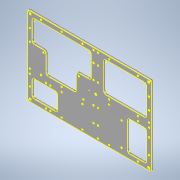
# Autodesk Inventor part: Platta
Saved by Autodesk Inventor 2021 (Build 250183000, 183)
## iProperties
Created: 2020-02-23
Part Number: Platta
Material: Generic
Document SubType Name: Modeling
Designer: lgnds
Density: 1 g/cm^3
Appearance: Default
Author: lgnds
Autodesk Inventor part; units mm, degrees
ref_plane "YZ Plane" through (0, 0, 0) normal (1, 0, 0) x (0, 1, 0)
ref_plane "XZ Plane" through (0, 0, 0) normal (0, 1, 0) x (-1, 0, 0)
ref_plane "Work Plane1" through (-121.526, 76.2535, 6) normal (0, 0, 1) x (1, 0, 0)
sketch "Sketch1" plane through (-121.526, 76.2535, 6) normal (0, 0, 1) x (1, 0, 0)
  line L0 (-3.6706, 3.4431) -> (246.7225, 3.4431)
  line L1 (246.7225, 3.4431) -> (246.7225, -155.95)
  line L2 (246.7225, -155.95) -> (-3.6706, -155.95)
  line L3 (-3.6706, -155.95) -> (-3.6706, 3.4431)
  line L4 (247.7225, -156.2501) -> (247.7225, 3.7432) projected
  line L5 (247.0226, -156.75) -> (-3.9707, -156.75) construction
  line L6 (247.0226, -156.75) -> (-3.9707, -156.75) projected
  line L7 (247.0226, 4.4431) -> (-3.9707, 4.4431) projected
  line L8 (247.0297, -157.8069) -> (-3.9777, -157.8069) projected
  ellipse E0 centre (247.0292, -156.2567) end of major axis (248.1256, -157.353) minor radius 1.55 (247.0297, -157.8069) -> (248.5794, -156.2572) ccw projected
  line L9 (248.5794, 3.7502) -> (248.5794, -156.2572) projected
  ellipse E1 centre (247.0292, 3.7498) end of major axis (248.1256, 4.8461) minor radius 1.55 (248.5794, 3.7502) -> (247.0297, 5.3) ccw projected
  line L10 (-3.9777, 5.3) -> (247.0297, 5.3) projected
  line L11 (-5.5275, -156.2572) -> (-5.5275, 3.7502) projected
  ellipse E2 centre (-3.9772, -156.2567) end of major axis (-5.0736, -157.353) minor radius 1.55 (-5.5275, -156.2572) -> (-3.9777, -157.8069) ccw projected
  ellipse E3 centre (-3.9705, 3.743) end of major axis (-4.4656, 4.2381) minor radius 0.7 (-3.9707, 4.4431) -> (-4.6706, 3.7432) ccw projected
  line L12 (247.0226, 4.4431) -> (-3.9707, 4.4431) projected
  ellipse E4 centre (247.0224, 3.743) end of major axis (247.5175, 4.2381) minor radius 0.7 (247.7225, 3.7432) -> (247.0226, 4.4431) ccw projected
  line L13 (247.7225, -156.2501) -> (247.7225, 3.7432) projected
  ellipse E5 centre (247.0224, -156.2499) end of major axis (247.5175, -156.745) minor radius 0.7 (247.0226, -156.95) -> (247.7225, -156.2501) ccw projected
  line L14 (-3.9707, -156.95) -> (247.0226, -156.95) projected
  line L15 (-4.6706, 3.7432) -> (-4.6706, -156.2501) projected
  line L16 (237.7225, -5.5569) -> (5.3294, -5.5569)
  line L17 (5.3294, -5.5569) -> (5.3294, -146.95)
  line L18 (5.3294, -146.95) -> (237.7225, -146.95)
  line L19 (237.7225, -146.95) -> (237.7225, -5.5569)
  ellipse E6 centre (-3.9772, 3.7498) end of major axis (-5.0736, 4.8461) minor radius 1.55 (-3.9777, 5.3) -> (-5.5275, 3.7502) ccw projected
  ellipse E7 centre (-3.9705, -156.2499) end of major axis (-4.4656, -156.745) minor radius 0.7 (-4.6706, -156.2501) -> (-3.9707, -156.95) ccw projected
  point P0 (121.526, -76.2535)
  dimension "d0" = 1
  dimension "d1" = 1
  dimension "d2" = 1
  dimension "d3" = 1
  dimension "d4" = 9
  constraints: 16 end point, 4 parallel, 2 perpendicular, 1 horizontal, 11 other
  measures "d0" distance between parallel lines of L7 L0
  measures "d1" distance between parallel lines of L15 L3
  measures "d2" distance between parallel lines of L4 L1
  measures "d3" distance between parallel lines of L14 L2
  measures "d4" distance between parallel lines of L0 L16
extrude "Extrusion1" add sketch "Sketch1" along normal blind 2.9864 contours L0 L1 L2 L3
sketch "Sketch2" plane through (-121.526, 76.2535, 8.9864) normal (0, 0, 1) x (1, 0, 0)
  circle A0 centre (1.526, -1.2535) radius 1.621 construction
  circle A1 centre (1.526, -151.2535) radius 1.621 construction
  circle A2 centre (241.526, -151.2535) radius 2.121 construction
  circle A3 centre (241.526, -1.2535) radius 2.121 construction
  circle A4 centre (1.526, -1.2535) radius 2.1
  line L0 (-92.7978, -76.2535) -> (335.0689, -76.2535) construction
  line L1 (121.526, -201.3727) -> (121.526, 48.8923) construction
  circle A5 centre (1.526, -151.2535) radius 1.621 construction
  circle A6 centre (1.526, -151.2535) radius 2.1
  circle A7 centre (241.526, -1.2535) radius 1.621 construction
  circle A8 centre (241.526, -151.2535) radius 1.621 construction
  circle A9 centre (241.526, -1.2535) radius 2.1
  circle A10 centre (241.526, -151.2535) radius 1.621 construction
  circle A11 centre (241.526, -151.2535) radius 2.1
  point P0 (121.526, -76.2535)
  point P1 (335.8498, -76.2535)
  dimension "d9" = 4.2
  constraints: 8 centre point, 8 symmetric about line, 4 coincident, 4 end point, 1 horizontal, 1 vertical, 11 other
  measures "d9" diameter of A4
extrude "Extrusion2" cut sketch "Sketch2" against normal up to next
sketch "Sketch3" plane through (-121.526, 76.2535, 8.9864) normal (0, 0, 1) x (1, 0, 0)
  line L0 (335.0689, -76.2535) -> (-92.7978, -76.2535) construction
  line L1 (5.3294, -81.2535) -> (237.7225, -81.2535)
  line L2 (237.7225, -81.2535) -> (237.7225, -71.2535)
  line L3 (237.7225, -71.2535) -> (5.3294, -71.2535)
  line L4 (5.3294, -71.2535) -> (5.3294, -81.2535)
  line L5 (5.3294, -81.2535) -> (237.7225, -71.2535) construction
  line L6 (237.7225, -81.2535) -> (5.3294, -71.2535) construction
  line L7 (5.3294, -146.95) -> (5.3294, -5.5569) construction
  point P0 (121.526, -76.2535)
  point P1 (5.3294, -76.2535)
  dimension "d10" = 10
  constraints: 14 end point, 4 midpoint, 2 horizontal, 2 parallel, 1 perpendicular, 2 other
  measures "d10" distance between parallel lines of L3 L1
extrude "Extrusion3" add sketch "Sketch3" against normal blind 2.9864
sketch "Sketch4" plane through (-121.526, 76.2535, 8.9864) normal (0, 0, 1) x (1, 0, 0)
  line L0 (-92.7978, -76.2535) -> (335.0689, -76.2535)
  line L1 (125.3294, -146.95) -> (135.3294, -146.95)
  line L2 (135.3294, -146.95) -> (135.3294, -5.5569)
  line L3 (135.3294, -5.5569) -> (125.3294, -5.5569)
  line L4 (125.3294, -5.5569) -> (125.3294, -146.95)
  line L5 (125.3294, -146.95) -> (135.3294, -5.5569) construction
  line L6 (135.3294, -146.95) -> (125.3294, -5.5569) construction
  line L7 (5.3294, -5.5569) -> (237.7225, -5.5569) projected
  line L8 (5.3294, -71.2535) -> (5.3294, -5.5569) projected
  point P0 (121.526, -76.2535)
  point P1 (130.3294, -76.2535)
  point P2 (130.3294, -5.5569)
  dimension "d13" = 10
  dimension "d14" = 120
  constraints: 14 end point, 3 midpoint, 2 horizontal, 2 parallel, 2 point on line, 1 perpendicular, 2 other
  measures "d13" distance between parallel lines of L2 L4
  measures "d14" distance between parallel lines of L8 L4
extrude "Extrusion4" add sketch "Sketch4" against normal blind 2.9864
fillet "Fillet1" radius 5 16 edges at (-116.1965, 70.6965, 7.4932) (3.8035, 70.6965, 7.4932) (3.8035, 5, 7.4932) (3.8035, -70.6965, 7.4932) (-116.1965, -70.6965, 7.4932) (3.8035, -5, 7.4932) (-116.1965, -5, 7.4932) (-116.1965, 5, 7.4932) (13.8035, -70.6965, 7.4932) (13.8035, -5, 7.4932) (13.8035, 70.6965, 7.4932) (116.1965, 70.6965, 7.4932) (116.1965, -5, 7.4932) (116.1965, -70.6965, 7.4932) (116.1965, 5, 7.4932) (13.8035, 5, 7.4932)
sketch "Sketch5" plane through (-121.526, 76.2535, 8.9864) normal (0, 0, 1) x (1, 0, 0)
  line L0 (-21.9579, -1.0569) -> (269.1636, -1.0569) construction
  circle A0 centre (1.526, -1.2535) radius 2.1 construction
  circle A1 centre (241.526, -1.2535) radius 2.1 construction
  circle A2 centre (23.3294, -1.0569) radius 1.6
  circle A3 centre (107.3294, -1.0569) radius 1.6
  circle A4 centre (161.3294, -1.0569) radius 1.6
  circle A5 centre (219.7225, -1.0569) radius 1.6
  line L1 (-165.7488, -76.2535) -> (448.2075, -76.2535) construction
  circle A6 centre (1.526, -151.2535) radius 2.1 construction
  circle A7 centre (241.526, -151.2535) radius 2.1 construction
  circle A8 centre (23.3294, -151.45) radius 1.6
  circle A9 centre (107.3294, -151.45) radius 1.6
  circle A10 centre (161.3294, -151.45) radius 1.6
  circle A11 centre (219.7225, -151.45) radius 1.6
  line L2 (5.3294, -66.2535) -> (5.3294, -10.5569) construction
  line L3 (125.3294, -10.5569) -> (125.3294, -66.2535) construction
  line L4 (135.3294, -66.2535) -> (135.3294, -10.5569) construction
  line L5 (237.7225, -10.5569) -> (237.7225, -66.2535) construction
  line L6 (130.3294, -1.0569) -> (130.3294, -154.6538) construction
  circle A12 centre (130.3294, -23.5569) radius 1.6 construction
  circle A13 centre (130.3294, -53.2535) radius 1.6 construction
  circle A14 centre (0.8294, -23.5569) radius 1.6
  circle A15 centre (0.8294, -53.2535) radius 1.6
  line L7 (10.3294, -5.5569) -> (120.3294, -5.5569) construction
  line L8 (120.3294, -71.2535) -> (10.3294, -71.2535) construction
  line L9 (121.526, 107.4883) -> (121.526, -256.8807) construction
  circle A16 centre (242.2225, -23.5569) radius 1.6
  circle A17 centre (242.2225, -53.2535) radius 1.6
  circle A18 centre (130.3294, -128.95) radius 1.6 construction
  circle A19 centre (130.3294, -99.2535) radius 1.6 construction
  circle A20 centre (0.8294, -128.95) radius 1.6 construction
  circle A21 centre (0.8294, -99.2535) radius 1.6 construction
  circle A22 centre (242.2225, -128.95) radius 1.6
  circle A23 centre (242.2225, -99.2535) radius 1.6
  line L10 (-48.6903, -38.6552) -> (287.1339, -38.6552) construction
  circle A24 centre (1.526, -76.0569) radius 2.1 construction
  circle A25 centre (23.3294, -76.2535) radius 1.6
  circle A26 centre (107.3294, -76.2535) radius 1.6
  circle A27 centre (161.3294, -76.2535) radius 1.6
  circle A28 centre (219.7225, -76.2535) radius 1.6
  line L11 (10.3294, -71.7535) -> (120.3294, -71.7535) construction
  line L12 (0.8294, 12.1079) -> (0.8294, -178.6983) construction
  line L13 (-3.6706, 3.4431) -> (-3.6706, -155.95) construction
  line L14 (65.3294, 41.7355) -> (65.3294, -183.4136) construction
  line L15 (176.0929, 55.4356) -> (176.0929, -204.828) construction
  line L16 (-78.0408, -113.8517) -> (360.4994, -113.8517) construction
  line L17 (246.7225, 3.4431) -> (-3.6706, 3.4431) projected
  point P0 (121.526, -76.2535)
  point P1 (-21.9579, -151.45)
  point P2 (5.3294, -86.2535)
  point P3 (125.3294, -86.2535)
  point P4 (135.3294, -86.2535)
  point P5 (237.7225, -86.2535)
  point P6 (5.3294, -66.7535)
  point P7 (125.3294, -66.7535)
  point P8 (135.3294, -66.7535)
  point P9 (130.3294, -76.2535)
  dimension "d18" = 3.2
  dimension "d19" = 3.2
  dimension "d20" = 3.2
  dimension "d21" = 3.2
  dimension "d22" = 18
  dimension "d23" = 18
  dimension "d24" = 26
  dimension "d25" = 18
  dimension "d26" = 10
  dimension "d27" = 5
  dimension "d28" = 3.2
  dimension "d29" = 3.2
  dimension "d30" = 3.2
  dimension "d31" = 3.2
  dimension "d32" = 18
  dimension "d33" = 18
  dimension "d34" = 18
  dimension "d35" = 18
  dimension "d36" = 37.5983
  dimension "d37" = 75.1965
  dimension "d40" = 4.5
  dimension "d41" = 9
  dimension "d48" = 37.5983
  dimension "d49" = 60
  dimension "d50" = 120
  dimension "d51" = 40.7634
  dimension "d52" = 102.3931
  dimension "d102" = 4.5
  constraints: 30 symmetric about line, 27 centre point, 16 end point, 9 point on line, 4 vertical, 3 horizontal, 19 other
  measures "d18" diameter of A2
  measures "d19" diameter of A3
  measures "d20" diameter of A4
  measures "d21" diameter of A5
  measures "d22" distance from line of L2 A2.centre
  measures "d23" distance from line of L3 A3.centre
  measures "d24" distance from line of L4 A4.centre
  measures "d25" distance from line of L5 A5.centre
  measures "d26" distance between parallel lines of L3 L4
  measures "d27" distance between parallel lines of L6 L4
  measures "d28" diameter of A13
  measures "d29" diameter of A12
  measures "d30" diameter of A14
  measures "d31" diameter of A15
  measures "d32" distance from line of L7 A14.centre
  measures "d33" distance from line of L8 A15.centre
  measures "d34" distance from line of L8 A13.centre
  measures "d35" distance from line of L7 A12.centre
  measures "d36" distance between parallel lines of L1 L10
  measures "d37" distance between parallel lines of L1 L0
  measures "d40" distance between parallel lines of L13 L12
  measures "d41" distance between parallel lines of L13 L2
  measures "d48" distance between parallel lines of L1 L16
  measures "d49" distance between parallel lines of L2 L14
  measures "d50" distance between parallel lines of L3 L2
  measures "d51" distance between parallel lines of L4 L15
  measures "d52" distance between parallel lines of L5 L4
  measures "d102" distance between parallel lines of L17 L0
extrude "Extrusion5" cut sketch "Sketch5" against normal up to next contours A2 | A3 | A4 | A5 | A8 | A9 | A10 | A11 | A14 | A15 | A16 | A17 | A22 | A25 | A26 | A27 | A28
sketch "Sketch6" plane through (-121.526, 76.2535, 8.9864) normal (0, 0, 1) x (1, 0, 0)
  line L0 (0.8294, -11.5974) -> (0.8294, -50.819) construction
  circle A0 centre (0.8294, -23.5569) radius 1.5 construction
  circle A1 centre (0.8294, -53.2535) radius 1.5 construction
  line L1 (121.526, 35.3217) -> (121.526, -187.8286) projected
  circle A2 centre (0.8294, -16.5569) radius 2
  circle A3 centre (0.8294, -60.5569) radius 2
  line L2 (242.2225, -11.5974) -> (242.2225, -50.819) construction
  circle A4 centre (242.2225, -23.5569) radius 1.5 construction
  circle A5 centre (242.2225, -53.2535) radius 1.5 construction
  circle A6 centre (242.2225, -16.5569) radius 2
  circle A7 centre (242.2225, -60.5569) radius 2
  point P0 (121.526, -76.2535)
  dimension "d42" = 4
  dimension "d43" = 4
  dimension "d44" = 44
  dimension "d45" = 7
  constraints: 8 point on line, 6 centre point, 6 symmetric about line, 4 end point, 1 vertical, 4 other
  measures "d42" diameter of A2
  measures "d43" diameter of A3
  measures "d44" distance of A2.centre A3.centre
  measures "d45" distance of A0.centre A2.centre
extrude "Extrusion6" [suppressed]
sketch "Sketch7" plane through (-121.526, 76.2535, 8.9864) normal (0, 0, 1) x (1, 0, 0)
  arc A0 (5.3294, -66.2535) -> (10.3294, -71.2535) centre (10.3294, -66.2535) ccw projected
  line L0 (5.3294, -66.2535) -> (125.3294, -66.2535)
  line L1 (125.3294, -66.2535) -> (125.3294, -86.2535)
  line L2 (125.3294, -86.2535) -> (5.3294, -86.2535)
  line L3 (5.3294, -86.2535) -> (5.3294, -66.2535)
  point P0 (121.526, -76.2535)
  constraints: 8 end point, 2 parallel, 1 horizontal, 1 perpendicular
extrude "Extrusion7" cut sketch "Sketch7" against normal up to next
sketch "Sketch8" plane through (-121.526, 76.2535, 8.9864) normal (0, 0, 1) x (1, 0, 0)
  line L0 (5.3294, -141.95) -> (5.3294, -10.5569) projected
  line L1 (125.3294, -141.95) -> (125.3294, -10.5569) projected
  line L2 (5.3294, -111.344) -> (125.3294, -111.344)
  line L3 (125.3294, -111.344) -> (125.3294, -93.344)
  line L4 (125.3294, -93.344) -> (5.3294, -93.344)
  line L5 (5.3294, -93.344) -> (5.3294, -111.344)
  line L6 (120.3294, -146.95) -> (10.3294, -146.95) projected
  line L7 (135.3294, -66.2535) -> (135.3294, -10.5569) projected
  line L8 (246.7225, -5.5569) -> (-3.6705, -5.5569) projected
  line L9 (140.3294, -5.5569) -> (232.7225, -5.5569) projected
  line L10 (143.3294, -5.5569) -> (135.3294, -5.5569)
  line L11 (135.3294, -5.5569) -> (135.3294, -146.95)
  line L12 (135.3294, -146.95) -> (143.3294, -146.95)
  line L13 (143.3294, -146.95) -> (143.3294, -5.5569)
  line L14 (232.7225, -146.95) -> (140.3294, -146.95) projected
  point P0 (121.526, -76.2535)
  dimension "d55" = 18
  dimension "d56" = 35.606
  dimension "d57" = 8
  dimension "d90" = 10
  constraints: 16 end point, 5 point on line, 4 parallel, 2 horizontal, 2 perpendicular
  measures "d55" distance between parallel lines of L4 L2
  measures "d56" distance between parallel lines of L6 L2
  measures "d57" distance between parallel lines of L7 L13
  measures "d90" distance between parallel lines of L11 L1
extrude "Extrusion8" add sketch "Sketch8" against normal up to surface (2.9864 mm away)
fillet "Fillet2" radius 5 8 edges at (21.8035, 70.6965, 7.4932) (21.8035, 5, 7.4932) (21.8035, -70.6965, 7.4932) (21.8035, -5, 7.4932) (3.8035, -35.0905, 7.4932) (3.8035, -17.0905, 7.4932) (-116.1965, -35.0905, 7.4932) (-116.1965, -17.0905, 7.4932)
sketch "Sketch9" plane through (-121.526, 76.2535, 8.9864) normal (0, 0, 1) x (1, 0, 0)
  circle A0 centre (0.8294, -53.2535) radius 1.5 construction
  circle A1 centre (1.526, -151.2535) radius 2.1 projected
  line L0 (0.8294, -53.2535) -> (0.8294, -142.4345) construction
  circle A2 centre (0.8294, -128.95) radius 1.6
  circle A3 centre (0.8294, -106.844) radius 1.6
  circle A4 centre (0.8294, -97.844) radius 1.6 construction
  line L1 (120.3294, -146.95) -> (10.3294, -146.95) construction
  circle A5 centre (23.3294, -151.45) radius 1.6 construction
  line L2 (5.3294, -141.95) -> (5.3294, -116.344) construction
  line L3 (10.3294, -111.344) -> (120.3294, -111.344) construction
  line L4 (120.3294, -93.344) -> (10.3294, -93.344) construction
  circle A6 centre (23.3294, -151.45) radius 1.6 construction
  circle A7 centre (107.3294, -151.45) radius 1.6 projected
  line L5 (23.3294, -151.45) -> (107.3294, -151.45) construction
  circle A8 centre (65.3294, -151.45) radius 1.6
  line L6 (131.159, -129.147) -> (47.2517, -129.147) construction
  line L7 (-44.2895, -102.344) -> (130.8356, -102.344) construction
  line L8 (120.3294, -111.344) -> (10.3294, -111.344) construction
  line L9 (23.3294, -106.844) -> (107.3294, -106.844) construction
  circle A9 centre (65.3294, -106.844) radius 1.6
  line L10 (10.3294, -93.344) -> (120.3294, -93.344) construction
  circle A10 centre (65.3294, -97.844) radius 1.6
  line L11 (23.3294, -97.844) -> (107.3294, -97.844) construction
  line L12 (120.3294, -93.344) -> (10.3294, -93.344) construction
  line L13 (65.3294, -97.844) -> (65.3294, -76.2535) construction
  circle A11 centre (129.8294, -128.95) radius 1.6
  circle A12 centre (129.8294, -106.844) radius 1.6 construction
  circle A13 centre (129.8294, -97.844) radius 1.6
  circle A14 centre (23.3294, -106.844) radius 1.6 construction
  circle A15 centre (23.3294, -106.844) radius 1.6 construction
  circle A16 centre (107.3294, -106.844) radius 1.6
  line L14 (10.3294, -93.344) -> (120.3294, -93.344) construction
  line L15 (23.3294, -97.844) -> (107.3294, -97.844) construction
  line L16 (120.3294, -93.344) -> (10.3294, -93.344) construction
  circle A17 centre (23.3294, -97.844) radius 1.6
  circle A18 centre (23.3294, -97.844) radius 1.6
  circle A19 centre (107.3294, -97.844) radius 1.6
  line L17 (134.3294, 25.9882) -> (134.3294, -179.8035) construction
  line L18 (125.3294, -10.5569) -> (125.3294, -88.344) construction
  line L19 (137.4999, -129.147) -> (221.4071, -129.147) construction
  circle A20 centre (138.8294, -128.95) radius 1.6
  circle A21 centre (138.8294, -97.844) radius 1.6
  circle A22 centre (0.8294, -23.5569) radius 1.5 projected
  circle A23 centre (0.8294, -53.2535) radius 1.5 projected
  circle A24 centre (129.8294, -53.2535) radius 1.5 construction
  circle A25 centre (129.8294, -23.5569) radius 1.5
  circle A26 centre (129.8294, -53.2535) radius 1.5
  circle A27 centre (138.8294, -53.2535) radius 1.5 construction
  circle A28 centre (138.8294, -23.5569) radius 1.5
  circle A29 centre (138.8294, -53.2535) radius 1.5
  line L20 (-36.5546, -49.4505) -> (71.8465, -49.4505) construction
  line L21 (10.3294, -5.5569) -> (120.3294, -5.5569) projected
  circle A30 centre (65.3294, -1.0569) radius 1.6
  circle A31 centre (33.3294, -106.844) radius 1.6
  line L22 (-44.2895, -155.95) -> (130.8356, -155.95) construction
  line L23 (23.3294, -151.45) -> (107.3294, -151.45) construction
  circle A32 centre (33.3294, -151.45) radius 1.6
  circle A33 centre (42.3294, -106.844) radius 1.6
  line L24 (10.3294, -146.95) -> (120.3294, -146.95) construction
  line L25 (23.3294, -151.45) -> (107.3294, -151.45) construction
  line L26 (120.3294, -146.95) -> (10.3294, -146.95) construction
  circle A34 centre (42.3294, -151.45) radius 1.6
  point P0 (121.526, -76.2535)
  point P1 (125.3294, -116.344)
  dimension "d61" = 3.2
  dimension "d62" = 3.2
  dimension "d63" = 3.2
  dimension "d64" = 18
  dimension "d65" = 18
  dimension "d66" = 4.5
  dimension "d67" = 4.5
  dimension "d68" = 3.2
  dimension "d69" = 42
  dimension "d70" = 84
  dimension "d71" = 17.803
  dimension "d72" = 35.606
  dimension "d73" = 9
  dimension "d74" = 9
  dimension "d77" = 43.8935
  dimension "d78" = 87.7871
  dimension "d79" = 3.2
  dimension "d80" = 28
  dimension "d83" = 3.2
  dimension "d84" = 9
  dimension "d152" = 3
  constraints: 42 end point, 28 centre point, 27 symmetric about line, 6 point on line, 4 horizontal, 3 vertical, 2 midpoint, 22 other
  measures "d61" diameter of A4
  measures "d62" diameter of A3
  measures "d63" diameter of A2
  measures "d64" distance from line of L1 A2.centre
  measures "d65" distance from line of A5.centre L2
  measures "d66" distance from line of L3 A3.centre
  measures "d67" distance from line of L4 A4.centre
  measures "d68" diameter of A8
  measures "d69" distance of A5.centre A8.centre
  measures "d70" distance of L5.end A5.centre
  measures "d71" distance between parallel lines of L1 L6
  measures "d72" distance between parallel lines of L1 L3
  measures "d73" distance between parallel lines of L7 L3
  measures "d74" distance between parallel lines of L18 L17
  measures "d77" distance between parallel lines of L4 L20
  measures "d78" distance between parallel lines of L14 L21
  measures "d79" diameter of A31
  measures "d80" distance from line of L2 A31.centre
  measures "d83" diameter of A33
  measures "d84" distance of A31.centre A33.centre
  measures "d152" diameter of A24
extrude "Extrusion9" cut sketch "Sketch9" against normal up to next contours A2 | A3 | A8 | A9 | A10 | A11 | A13 | A16 | A17 | A19 | A20 | A21 | A22 | A23 | A25 | A26 | A28 | A29 | A30 | A31 | A32 | A33 | A34
sketch "Sketch10" plane through (-121.526, 76.2535, 8.9864) normal (0, 0, 1) x (1, 0, 0)
  circle A0 centre (23.3294, -151.2535) radius 1.5 construction
  circle A1 centre (23.3294, -151.45) radius 1.6 projected
  point P0 (121.526, -76.2535)
extrude "Extrusion10" add sketch "Sketch10" against normal up to surface (2.9864 mm away)
sketch "Sketch11" plane through (-121.526, 76.2535, 8.9864) normal (0, 0, 1) x (1, 0, 0)
  arc A0 (143.3294, -66.2535) -> (148.3294, -71.2535) centre (148.3294, -66.2535) ccw projected
  line L0 (237.7225, -86.2535) -> (237.7225, -141.95) projected
  line L1 (143.3294, -66.2535) -> (237.7225, -66.2535)
  line L2 (237.7225, -66.2535) -> (237.7225, -86.2535)
  line L3 (237.7225, -86.2535) -> (143.3294, -86.2535)
  line L4 (143.3294, -86.2535) -> (143.3294, -66.2535)
  point P0 (121.526, -76.2535)
  constraints: 8 end point, 2 parallel, 1 horizontal, 1 perpendicular
extrude "Extrusion11" cut sketch "Sketch11" against normal up to surface (2.9864 mm away)
sketch "Sketch12" plane through (-121.526, 76.2535, 8.9864) normal (0, 0, 1) x (1, 0, 0)
  line L0 (143.3294, -141.95) -> (143.3294, -10.5569) projected
  line L1 (237.7225, -10.5569) -> (237.7225, -141.95) projected
  line L2 (-53.7492, -76.2535) -> (296.8011, -76.2535) construction
  line L3 (143.3294, -85.2535) -> (237.7225, -85.2535)
  line L4 (237.7225, -85.2535) -> (237.7225, -67.2535)
  line L5 (237.7225, -67.2535) -> (143.3294, -67.2535)
  line L6 (143.3294, -67.2535) -> (143.3294, -85.2535)
  line L7 (143.3294, -85.2535) -> (237.7225, -67.2535) construction
  line L8 (237.7225, -85.2535) -> (143.3294, -67.2535) construction
  line L9 (125.3294, -10.5569) -> (125.3294, -88.344) projected
  line L10 (120.3294, -93.344) -> (10.3294, -93.344) projected
  line L11 (10.3294, -111.344) -> (120.3294, -111.344) projected
  line L12 (143.3294, -141.95) -> (143.3294, -10.5569) projected
  line L13 (143.3294, -71.7535) -> (237.7225, -71.7535) construction
  circle A0 centre (161.3294, -71.7535) radius 1.6
  circle A1 centre (219.7225, -71.7535) radius 1.6
  circle A2 centre (161.3294, -1.0569) radius 1.6 projected
  circle A3 centre (161.3294, -80.7535) radius 1.6
  circle A4 centre (219.7225, -80.7535) radius 1.6
  point P0 (121.526, -76.2535)
  point P1 (190.526, -76.2535)
  dimension "d87" = 18
  dimension "d88" = 18
  dimension "d89" = 18
  dimension "d91" = 4.5
  dimension "d92" = 18
  dimension "d93" = 18
  dimension "d94" = 18
  dimension "d95" = 3.2
  dimension "d96" = 3.2
  dimension "d97" = 3.2
  constraints: 14 end point, 7 point on line, 4 centre point, 2 midpoint, 2 parallel, 2 perpendicular, 2 symmetric about line, 1 horizontal, 2 other
  measures "d87" distance between parallel lines of L5 L3
  measures "d88" distance between parallel lines of L9 L0
  measures "d89" distance between parallel lines of L10 L11
  measures "d91" distance between parallel lines of L5 L13
  measures "d92" distance from line of L0 A0.centre
  measures "d93" distance from line of L0 A2.centre
  measures "d94" distance from line of L1 A1.centre
  measures "d95" diameter of A2
  measures "d96" diameter of A0
  measures "d97" diameter of A1
extrude "Extrusion12" add sketch "Sketch12" against normal up to surface (2.9864 mm away) contours L0 L5 L1 L3
fillet "Fillet3" radius 5 4 edges at (21.8035, -9, 7.4932) (21.8035, 9, 7.4932) (116.1965, 9, 7.4932) (116.1965, -9, 7.4932)
fillet "Fillet4" radius 2 4 edges at (125.1965, -79.6965, 7.4932) (125.1965, 79.6965, 7.4932) (-125.1965, 79.6965, 7.4932) (-125.1965, -79.6965, 7.4932)
sketch "Sketch13" plane through (-121.526, 76.2535, 8.9864) normal (0, 0, 1) x (1, 0, 0)
  circle A0 centre (138.8294, -97.844) radius 1.6 projected
  line L0 (138.8294, -97.844) -> (272.4604, -97.844) construction
  circle A1 centre (242.2225, -53.2535) radius 1.6 projected
  line L1 (242.2225, -53.2535) -> (242.2225, -126.2717) construction
  circle A2 centre (242.2225, -97.844) radius 1.6
  point P0 (121.526, -76.2535)
  dimension "d103" = 3.2
  constraints: 4 end point, 2 point on line, 1 centre point, 1 horizontal, 1 vertical
  measures "d103" diameter of A2
extrude "Extrusion13" cut sketch "Sketch13" against normal blind 10 contours A2
sketch "Sketch14" plane through (-121.526, 76.2535, 8.9864) normal (0, 0, 1) x (1, 0, 0)
  line L0 (10.3294, -5.5569) -> (120.3294, -5.5569) projected
  circle A0 centre (0.8294, -23.5569) radius 1.6 projected
  line L1 (120.3294, -93.344) -> (10.3294, -93.344) projected
  circle A1 centre (0.8294, -53.2535) radius 1.6 projected
  circle A2 centre (0.8294, -60.5569) radius 2 projected
  circle A3 centre (0.8294, -16.5569) radius 2 projected
  circle A4 centre (242.2225, -23.5569) radius 1.6 projected
  circle A5 centre (242.2225, -53.2535) radius 1.6 projected
  point P0 (121.526, -76.2535)
  dimension "d106" = 18
  dimension "d107" = 40.0905
  dimension "d108" = 7.3035
  dimension "d109" = 7
  measures "d106" distance from line of L0 A0.centre
  measures "d107" distance from line of L1 A1.centre
  measures "d108" distance of A1.centre A2.centre
  measures "d109" distance of A3.centre A0.centre
extrude "Extrusion14" add sketch "Sketch14" against normal up to surface (2.9864 mm away) contours A0 | A1 | A4 | A5
sketch "Sketch15" plane through (-121.526, 76.2535, 8.9864) normal (0, 0, 1) x (1, 0, 0)
  circle A0 centre (0.8294, -106.844) radius 1.6 projected
  line L0 (0.8294, -106.844) -> (0.8294, 12.462) construction
  circle A1 centre (0.8294, -50.5569) radius 1.6
  circle A2 centre (0.8294, -26.5569) radius 1.6
  line L1 (10.3294, -5.5569) -> (120.3294, -5.5569) projected
  circle A3 centre (23.3294, -1.0569) radius 1.6 projected
  circle A4 centre (0.8294, -16.5569) radius 2 projected
  circle A5 centre (0.8294, -60.5569) radius 2 projected
  line L2 (121.526, 46.1444) -> (121.526, -189.6324) projected
  circle A6 centre (242.2225, -50.5569) radius 1.6
  circle A7 centre (242.2225, -26.5569) radius 1.6
  point P0 (121.526, -76.2535)
  dimension "d112" = 21
  dimension "d113" = 3.2
  dimension "d114" = 3.2
  dimension "d115" = 10
  dimension "d116" = 10
  dimension "d117" = 3.2
  constraints: 4 centre point, 2 end point, 2 point on line, 2 symmetric about line, 1 vertical, 2 other
  measures "d112" distance from line of L1 A2.centre
  measures "d113" diameter of A2
  measures "d114" diameter of A3
  measures "d115" distance of A4.centre A2.centre
  measures "d116" distance of A5.centre A1.centre
  measures "d117" diameter of A1
extrude "Extrusion15" cut sketch "Sketch15" against normal blind 10 contours A1 | A2 | A6 | A7
sketch "Sketch16" plane through (-121.526, 76.2535, 8.9864) normal (0, 0, 1) x (1, 0, 0)
  circle A0 centre (107.3294, -1.0569) radius 1.6 construction
  circle A1 centre (129.8294, -23.5569) radius 1.5 construction
  circle A2 centre (138.8294, -23.5569) radius 1.5 construction
  circle A3 centre (161.3294, -1.0569) radius 1.6 construction
  line L0 (107.3294, -1.0569) -> (161.3294, -1.0569) construction
  line L1 (129.8294, -23.5569) -> (129.8294, -1.0569) construction
  line L2 (138.8294, -23.5569) -> (138.8294, -1.0569) construction
  circle A4 centre (138.8294, -128.95) radius 1.6 construction
  circle A5 centre (161.3294, -151.45) radius 1.6 construction
  circle A6 centre (138.8294, -128.95) radius 1.6 construction
  line L3 (138.8294, -128.95) -> (138.8294, -151.45) construction
  line L4 (138.8294, -151.45) -> (161.3294, -151.45) construction
  circle A7 centre (219.7225, -80.7535) radius 1.6 construction
  circle A8 centre (242.2225, -97.844) radius 1.6 construction
  circle A9 centre (219.7225, -71.7535) radius 1.6 construction
  line L5 (242.2225, -97.844) -> (242.2225, -66.5616) construction
  line L6 (219.7225, -80.7535) -> (242.2225, -80.7535) construction
  line L7 (219.7225, -71.7535) -> (242.2225, -71.7535) construction
  circle A10 centre (0.8294, -50.5569) radius 1.6 construction
  circle A11 centre (23.3294, -97.844) radius 1.6 construction
  circle A12 centre (23.3294, -97.844) radius 1.6 construction
  line L8 (23.3294, -97.844) -> (0.8294, -97.844) construction
  line L9 (0.8294, -97.844) -> (0.8294, -50.5569) construction
  circle A13 centre (129.8294, -1.0569) radius 1.6
  circle A14 centre (138.8294, -1.0569) radius 1.6
  circle A15 centre (242.2225, -71.7535) radius 1.6
  circle A16 centre (242.2225, -80.7535) radius 1.6
  circle A17 centre (138.8294, -151.45) radius 1.6
  circle A18 centre (0.8294, -97.844) radius 1.6
  line L10 (134.3294, -1.0569) -> (134.3294, -91.3171) construction
  line L11 (242.2225, -76.2535) -> (134.3294, -76.2535) construction
  circle A19 centre (134.3294, -76.2535) radius 2.1
  circle A20 centre (241.526, -1.2535) radius 2.1 construction
  point P0 (121.526, -76.2535)
  dimension "d120" = 4.5
  dimension "d121" = 9
  dimension "d122" = 4.2
  dimension "d123" = 3.2
  dimension "d124" = 3.2
  dimension "d125" = 3.2
  dimension "d126" = 3.2
  dimension "d127" = 3.2
  dimension "d128" = 3.2
  dimension "d129" = 3.2
  dimension "d130" = 4.2
  constraints: 24 end point, 7 centre point, 7 coincident, 6 point on line, 5 perpendicular, 4 horizontal, 3 vertical, 1 midpoint
  measures "d120" distance between parallel lines of L11 L7
  measures "d121" distance between parallel lines of L7 L6
  measures "d122" diameter of A20
  measures "d123" diameter of A13
  measures "d124" diameter of A3
  measures "d125" diameter of A14
  measures "d126" diameter of A15
  measures "d127" diameter of A16
  measures "d128" diameter of A17
  measures "d129" diameter of A18
  measures "d130" diameter of A19
extrude "Extrusion16" cut sketch "Sketch16" against normal up to next
sketch "Sketch17" plane through (-121.526, 76.2535, 6) normal (0, 0, -1) x (-1, 0, 0)
  arc A0 (-143.3294, -10.5569) -> (-148.3294, -5.5569) centre (-148.3294, -10.5569) ccw projected
  arc A1 (-148.3294, -67.2535) -> (-143.3294, -62.2535) centre (-148.3294, -62.2535) ccw projected
  line L0 (-143.3294, -62.2535) -> (-143.3294, -10.5569) projected
  line L1 (-232.7225, -5.5569) -> (-148.3294, -5.5569) projected
  line L2 (-232.7225, -67.2535) -> (-148.3294, -67.2535) projected
  line L3 (-150.3294, -5.5569) -> (-150.3294, -67.2535)
  point P0 (-121.526, -76.2535)
  dimension "d133" = 7
  constraints: 2 end point, 2 point on line, 1 perpendicular
  measures "d133" distance between parallel lines of L0 L3
extrude "Extrusion17" add sketch "Sketch17" against normal up to surface (2.9864 mm away)
sketch "Sketch18" plane through (-121.526, 76.2535, 6) normal (0, 0, -1) x (-1, 0, 0)
  line L0 (-143.3294, -141.95) -> (-143.3294, -90.2535) projected
  arc A0 (-143.3294, -90.2535) -> (-148.3294, -85.2535) centre (-148.3294, -90.2535) ccw projected
  line L1 (-148.3294, -85.2535) -> (-232.7225, -85.2535) projected
  arc A1 (-148.3294, -146.95) -> (-143.3294, -141.95) centre (-148.3294, -141.95) ccw projected
  line L2 (-148.3294, -146.95) -> (-232.7225, -146.95) projected
  line L3 (-148.3294, -85.2535) -> (-232.7225, -85.2535) projected
  line L4 (-198.3294, -85.2535) -> (-198.3294, -146.95)
  point P0 (-121.526, -76.2535)
  dimension "d136" = 55
  constraints: 2 end point, 2 point on line, 1 perpendicular
  measures "d136" distance between parallel lines of L0 L4
extrude "Extrusion18" add sketch "Sketch18" against normal up to surface (2.9864 mm away)
sketch "Sketch19" plane through (-121.526, 76.2535, 6) normal (0, 0, -1) x (-1, 0, 0)
  line L0 (-125.3294, -141.95) -> (-125.3294, -116.344) projected
  arc A0 (-120.3294, -111.344) -> (-125.3294, -116.344) centre (-120.3294, -116.344) ccw projected
  line L1 (-10.3294, -111.344) -> (-120.3294, -111.344) projected
  arc A1 (-125.3294, -141.95) -> (-120.3294, -146.95) centre (-120.3294, -141.95) ccw projected
  line L2 (-10.3294, -146.95) -> (-120.3294, -146.95) projected
  line L3 (-10.3294, -111.344) -> (-120.3294, -111.344) projected
  line L4 (-57.3294, -111.344) -> (-57.3294, -146.95)
  point P0 (-121.526, -76.2535)
  dimension "d139" = 68
  constraints: 2 end point, 2 point on line, 1 perpendicular
  measures "d139" distance between parallel lines of L0 L4
extrude "Extrusion19" add sketch "Sketch19" against normal up to surface (2.9864 mm away)
sketch "Sketch20" plane through (-121.526, 76.2535, 6) normal (0, 0, -1) x (-1, 0, 0)
  line L0 (-125.3294, -88.344) -> (-125.3294, -10.5569) projected
  arc A0 (-125.3294, -88.344) -> (-120.3294, -93.344) centre (-120.3294, -88.344) ccw projected
  line L1 (-120.3294, -93.344) -> (-10.3294, -93.344) projected
  line L2 (-125.3294, -10.5569) -> (-125.3294, -88.344) projected
  line L3 (-125.3294, -56.344) -> (-95.3294, -56.344)
  line L4 (-95.3294, -56.344) -> (-95.3294, -93.344)
  arc A1 (-10.3294, -93.344) -> (-5.3294, -88.344) centre (-10.3294, -88.344) ccw projected
  line L5 (-5.3294, -10.5569) -> (-5.3294, -88.344) projected
  line L6 (-5.3294, -88.344) -> (-5.3294, -10.5569) projected
  line L7 (-5.3294, -51.344) -> (-33.3294, -51.344)
  line L8 (-33.3294, -51.344) -> (-33.3294, -93.344)
  point P0 (-121.526, -76.2535)
  dimension "d142" = 37
  dimension "d143" = 30
  dimension "d146" = 28
  dimension "d180" = 42
  constraints: 8 end point, 4 point on line, 3 perpendicular, 1 horizontal
  measures "d142" distance between parallel lines of L1 L3
  measures "d143" distance between parallel lines of L0 L4
  measures "d146" distance between parallel lines of L5 L8
  measures "d180" distance between parallel lines of L1 L7
extrude "Extrusion20" add sketch "Sketch20" against normal up to surface (2.9864 mm away)
fillet "Fillet5" radius 5 12 edges at (28.8035, 70.6965, 7.4932) (28.8035, 9, 7.4932) (76.8035, -9, 7.4932) (76.8035, -70.6965, 7.4932) (3.8035, 19.9095, 7.4932) (-26.1965, -17.0905, 7.4932) (-88.1965, -17.0905, 7.4932) (-26.1965, 19.9095, 7.4932) (-88.1965, 24.9095, 7.4932) (-116.1965, 24.9095, 7.4932) (-64.1965, -35.0905, 7.4932) (-64.1965, -70.6965, 7.4932)
sketch "Sketch22" plane through (-121.526, 76.2535, 8.9864) normal (0, 0, 1) x (1, 0, 0)
  circle A0 centre (138.8294, -53.2535) radius 1.5 construction
  circle A1 centre (129.8294, -53.2535) radius 1.5 construction
  circle A2 centre (138.8294, -23.5569) radius 1.5 construction
  circle A3 centre (129.8294, -23.5569) radius 1.5 construction
  circle A4 centre (138.8294, -53.2535) radius 1.6
  circle A5 centre (129.8294, -53.2535) radius 1.6
  circle A6 centre (129.8294, -23.5569) radius 1.6
  circle A7 centre (138.8294, -23.5569) radius 1.6
  circle A8 centre (161.3294, -71.7535) radius 1.6 projected
  point P0 (121.526, -76.2535)
  dimension "d153" = 3.2
  dimension "d154" = 3.2
  dimension "d155" = 3.2
  dimension "d156" = 3.2
  dimension "d157" = 3.2
  constraints: 4 centre point
  measures "d153" diameter of A8
  measures "d154" diameter of A4
  measures "d155" diameter of A5
  measures "d156" diameter of A7
  measures "d157" diameter of A6
extrude "Extrusion21" cut sketch "Sketch22" against normal blind 10 contours A4 | A5 | A6 | A7
sketch "Sketch23" plane through (-121.526, 76.2535, 6) normal (0, 0, -1) x (-1, 0, 0)
  arc A0 (-95.3294, -61.344) -> (-100.3294, -56.344) centre (-100.3294, -61.344) ccw projected
  arc A1 (-28.3294, -51.344) -> (-33.3294, -56.344) centre (-28.3294, -56.344) ccw projected
  circle A2 centre (-100.3294, -61.344) radius 1.6
  circle A3 centre (-28.3294, -56.344) radius 1.6
  circle A4 centre (-129.8294, -53.2535) radius 1.6 projected
  circle A5 centre (-161.3294, -80.7535) radius 1.6 construction
  circle A6 centre (-161.3294, -151.45) radius 1.6 construction
  circle A7 centre (-186.7225, -143.95) radius 1.6
  line L0 (-246.7225, 1.4431) -> (-246.7225, -153.95) projected
  line L1 (-244.7225, -155.95) -> (1.6706, -155.95) projected
  line L2 (-186.7225, -143.95) -> (-186.7225, -80.7535) construction
  circle A8 centre (-186.7225, -95.95) radius 1.6
  point P0 (-121.526, -76.2535)
  dimension "d160" = 3.2
  dimension "d161" = 3.2
  dimension "d162" = 3.2
  dimension "d165" = 3.2
  dimension "d169" = 60
  dimension "d170" = 12
  dimension "d171" = 48
  dimension "d172" = 3.2
  constraints: 4 centre point, 2 coincident, 2 end point, 1 point on line, 1 vertical
  measures "d160" diameter of A2
  measures "d161" diameter of A4
  measures "d162" diameter of A3
  measures "d165" diameter of A7
  measures "d169" distance from line of L0 L2.start
  measures "d170" distance from line of L1 L2.start
  measures "d171" distance of L2.start A8.centre
  measures "d172" diameter of A8
extrude "Extrusion22" cut sketch "Sketch23" against normal blind 10 contours A2 | A3 | A7 | A8
sketch "Sketch24" plane through (-121.526, 76.2535, 8.9864) normal (0, 0, 1) x (1, 0, 0)
  circle A0 centre (107.3294, -97.844) radius 1.6 projected
  point P0 (121.526, -76.2535)
extrude "Extrusion23" add sketch "Sketch24" against normal up to surface (2.9864 mm away)
sketch "Sketch25" plane through (-121.526, 76.2535, 8.9864) normal (0, 0, 1) x (1, 0, 0)
  circle A0 centre (65.3294, -97.844) radius 1.6 projected
  circle A1 centre (129.8294, -97.844) radius 1.6 projected
  circle A2 centre (65.3294, -97.844) radius 1.6 projected
  line L0 (65.3294, -97.844) -> (129.8294, -97.844)
  circle A3 centre (109.3294, -97.844) radius 1.6
  circle A4 centre (107.3294, -106.844) radius 1.6 projected
  point P0 (121.526, -76.2535)
  dimension "d175" = 3.2
  dimension "d176" = 3.2
  dimension "d177" = 2
  constraints: 2 end point, 1 centre point, 1 horizontal, 1 point on line
  measures "d175" diameter of A0
  measures "d176" diameter of A3
  measures "d177" horizontal distance of A3.centre A4.centre
extrude "Extrusion24" cut sketch "Sketch25" against normal through all contours A3 L0 | L0 A3
sketch "Sketch26" plane through (-121.526, 76.2535, 8.9864) normal (0, 0, 1) x (1, 0, 0)
  circle A0 centre (109.3294, -97.844) radius 1.6 projected
  circle A1 centre (186.7225, -143.95) radius 1.6 projected
  circle A2 centre (100.3294, -61.344) radius 1.6 projected
  circle A3 centre (28.3294, -56.344) radius 1.6 projected
  circle A4 centre (186.7225, -95.95) radius 1.6 projected
  circle A5 centre (129.8294, -23.5569) radius 1.6 projected
  circle A6 centre (138.8294, -53.2535) radius 1.6 projected
  circle A7 centre (129.8294, -53.2535) radius 1.6 projected
  circle A8 centre (138.8294, -23.5569) radius 1.6 projected
  arc A9 (33.3294, -56.344) -> (28.3294, -51.344) centre (28.3294, -56.344) ccw projected
  line L0 (10.3294, -51.344) -> (28.3294, -51.344) projected
  arc A10 (5.3294, -46.344) -> (10.3294, -51.344) centre (10.3294, -46.344) ccw projected
  line L1 (5.3294, -46.344) -> (5.3294, -10.5569) projected
  arc A11 (10.3294, -5.5569) -> (5.3294, -10.5569) centre (10.3294, -10.5569) ccw projected
  line L2 (10.3294, -5.5569) -> (120.3294, -5.5569) projected
  arc A12 (125.3294, -10.5569) -> (120.3294, -5.5569) centre (120.3294, -10.5569) ccw projected
  line L3 (125.3294, -10.5569) -> (125.3294, -51.344) projected
  arc A13 (120.3294, -56.344) -> (125.3294, -51.344) centre (120.3294, -51.344) ccw projected
  line L4 (100.3294, -56.344) -> (120.3294, -56.344) projected
  arc A14 (100.3294, -56.344) -> (95.3294, -61.344) centre (100.3294, -61.344) ccw projected
  line L5 (95.3294, -88.344) -> (95.3294, -61.344) projected
  arc A15 (90.3294, -93.344) -> (95.3294, -88.344) centre (90.3294, -88.344) ccw projected
  line L6 (90.3294, -93.344) -> (38.3294, -93.344) projected
  arc A16 (33.3294, -88.344) -> (38.3294, -93.344) centre (38.3294, -88.344) ccw projected
  line L7 (33.3294, -56.344) -> (33.3294, -88.344) projected
  circle A17 centre (0.8294, -97.844) radius 1.6 projected
  circle A18 centre (242.2225, -80.7535) radius 1.6 projected
  circle A19 centre (138.8294, -1.0569) radius 1.6 projected
  circle A20 centre (129.8294, -1.0569) radius 1.6 projected
  circle A21 centre (242.2225, -71.7535) radius 1.6 projected
  circle A22 centre (138.8294, -151.45) radius 1.6 projected
  circle A23 centre (134.3294, -76.2535) radius 2.1 projected
  circle A24 centre (242.2225, -50.5569) radius 1.6 projected
  circle A25 centre (0.8294, -50.5569) radius 1.6 projected
  circle A26 centre (0.8294, -26.5569) radius 1.6 projected
  circle A27 centre (242.2225, -26.5569) radius 1.6 projected
  circle A28 centre (242.2225, -97.844) radius 1.6 projected
  arc A29 (-3.6706, -153.95) -> (-1.6706, -155.95) centre (-1.6706, -153.95) ccw projected
  line L8 (-1.6706, -155.95) -> (244.7225, -155.95) projected
  arc A30 (244.7225, -155.95) -> (246.7225, -153.95) centre (244.7225, -153.95) ccw projected
  line L9 (246.7225, -153.95) -> (246.7225, 1.4431) projected
  arc A31 (246.7225, 1.4431) -> (244.7225, 3.4431) centre (244.7225, 1.4431) ccw projected
  line L10 (244.7225, 3.4431) -> (-1.6706, 3.4431) projected
  arc A32 (-1.6706, 3.4431) -> (-3.6706, 1.4431) centre (-1.6706, 1.4431) ccw projected
  line L11 (-3.6706, 1.4431) -> (-3.6706, -153.95) projected
  circle A33 centre (42.3294, -106.844) radius 1.6 projected
  circle A34 centre (33.3294, -106.844) radius 1.6 projected
  circle A35 centre (138.8294, -128.95) radius 1.6 projected
  circle A36 centre (107.3294, -106.844) radius 1.6 projected
  circle A37 centre (129.8294, -128.95) radius 1.6 projected
  circle A38 centre (65.3294, -106.844) radius 1.6 projected
  circle A39 centre (0.8294, -106.844) radius 1.6 projected
  circle A40 centre (0.8294, -128.95) radius 1.6 projected
  circle A41 centre (65.3294, -151.45) radius 1.6 projected
  circle A42 centre (65.3294, -97.844) radius 1.6 projected
  circle A43 centre (129.8294, -97.844) radius 1.6 projected
  circle A44 centre (23.3294, -97.844) radius 1.6 projected
  circle A45 centre (138.8294, -97.844) radius 1.6 projected
  circle A46 centre (65.3294, -1.0569) radius 1.6 projected
  circle A47 centre (33.3294, -151.45) radius 1.6 projected
  circle A48 centre (42.3294, -151.45) radius 1.6 projected
  line L12 (52.3294, -146.95) -> (10.3294, -146.95) projected
  arc A49 (5.3294, -141.95) -> (10.3294, -146.95) centre (10.3294, -141.95) ccw projected
  line L13 (5.3294, -141.95) -> (5.3294, -116.344) projected
  arc A50 (10.3294, -111.344) -> (5.3294, -116.344) centre (10.3294, -116.344) ccw projected
  line L14 (10.3294, -111.344) -> (52.3294, -111.344) projected
  arc A51 (57.3294, -116.344) -> (52.3294, -111.344) centre (52.3294, -116.344) ccw projected
  line L15 (57.3294, -141.95) -> (57.3294, -116.344) projected
  arc A52 (52.3294, -146.95) -> (57.3294, -141.95) centre (52.3294, -141.95) ccw projected
  line L16 (203.3294, -85.2535) -> (232.7225, -85.2535) projected
  arc A53 (237.7225, -90.2535) -> (232.7225, -85.2535) centre (232.7225, -90.2535) ccw projected
  line L17 (237.7225, -90.2535) -> (237.7225, -141.95) projected
  arc A54 (232.7225, -146.95) -> (237.7225, -141.95) centre (232.7225, -141.95) ccw projected
  line L18 (232.7225, -146.95) -> (203.3294, -146.95) projected
  arc A55 (198.3294, -141.95) -> (203.3294, -146.95) centre (203.3294, -141.95) ccw projected
  line L19 (198.3294, -90.2535) -> (198.3294, -141.95) projected
  arc A56 (203.3294, -85.2535) -> (198.3294, -90.2535) centre (203.3294, -90.2535) ccw projected
  circle A57 centre (241.526, -1.2535) radius 2.1 projected
  circle A58 centre (1.526, -1.2535) radius 2.1 projected
  circle A59 centre (1.526, -151.2535) radius 2.1 projected
  circle A60 centre (241.526, -151.2535) radius 2.1 projected
  circle A61 centre (242.2225, -128.95) radius 1.6 projected
  circle A62 centre (161.3294, -151.45) radius 1.6 projected
  circle A63 centre (161.3294, -1.0569) radius 1.6 projected
  circle A64 centre (23.3294, -1.0569) radius 1.6 projected
  circle A65 centre (107.3294, -1.0569) radius 1.6 projected
  circle A66 centre (219.7225, -1.0569) radius 1.6 projected
  circle A67 centre (107.3294, -151.45) radius 1.6 projected
  circle A68 centre (219.7225, -151.45) radius 1.6 projected
  circle A69 centre (161.3294, -80.7535) radius 1.6 projected
  circle A70 centre (219.7225, -80.7535) radius 1.6 projected
  circle A71 centre (219.7225, -71.7535) radius 1.6 projected
  circle A72 centre (161.3294, -71.7535) radius 1.6 projected
  line L20 (155.3294, -5.5569) -> (232.7225, -5.5569) projected
  arc A73 (237.7225, -10.5569) -> (232.7225, -5.5569) centre (232.7225, -10.5569) ccw projected
  line L21 (237.7225, -10.5569) -> (237.7225, -62.2535) projected
  arc A74 (232.7225, -67.2535) -> (237.7225, -62.2535) centre (232.7225, -62.2535) ccw projected
  line L22 (232.7225, -67.2535) -> (155.3294, -67.2535) projected
  arc A75 (150.3294, -62.2535) -> (155.3294, -67.2535) centre (155.3294, -62.2535) ccw projected
  line L23 (150.3294, -10.5569) -> (150.3294, -62.2535) projected
  arc A76 (155.3294, -5.5569) -> (150.3294, -10.5569) centre (155.3294, -10.5569) ccw projected
  point P0 (121.526, -76.2535)
equation "\"d1\" = d0"
equation "\"d2\" = d1"
equation "\"d3\" = d2"
equation "\"d11\" = d5"
equation "\"d15\" = d11"
equation "\"d19\" = d18"
equation "\"d20\" = d18"
equation "\"d21\" = d18"
equation "\"d23\" = d22"
equation "\"d27\" = 0.5 * d26"
equation "\"d28\" = d18"
equation "\"d29\" = d18"
equation "\"d30\" = d18"
equation "\"d31\" = d18"
equation "\"d32\" = d22"
equation "\"d33\" = d22"
equation "\"d34\" = d33"
equation "\"d35\" = d22"
equation "\"d36\" = 0.5 * d37"
equation "\"d40\" = 0.5 * d41"
equation "\"d48\" = d36"
equation "\"d49\" = 0.5 * d50"
equation "\"d43\" = d42"
equation "\"d5\" = 2.986356"
body "Solid1"
